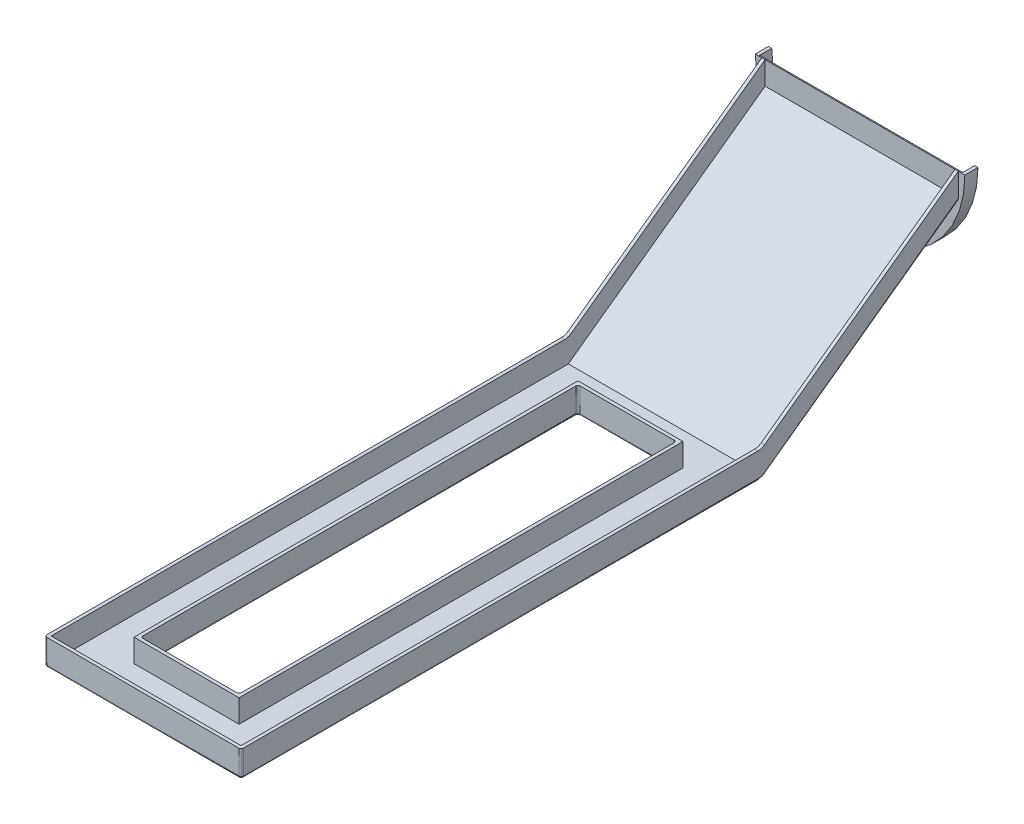
# Autodesk Inventor part: TYLNA SZARA OBUDOWA STOJAKA
Saved by Autodesk Inventor 2017 SP1 (Build 210196100, 196)
## iProperties
Created: 2020-12-26
Part Number: TYLNA SZARA OBUDOWA STOJAKA
Material: Tworzywo sztuczne, nieprzezroczyste czarne
Document SubType Name: Modeling
Designer: Napoleon
Mass: 96.6622 g
Surface Area: 795.491 cm^2
Volume: 101.536 cm^3
Density: 0.952 g/cm^3
Appearance: Teksturowany — drobny — czarny
Author: Napoleon
Autodesk Inventor part; units mm, degrees
ref_plane "YZ Plane" through (0, 0, 0) normal (1, 0, 0) x (0, 1, 0)
sketch "Szkic1" plane through (0, 0, 0) normal (0, 0, 1) x (1, 0, 0)
  line L0 (-44.8776, 28.0247) -> (-44.8776, 13.0664) projected
  arc A0 (-44.8776, 13.0664) -> (-35.2734, -8.1745) centre (0, 20.5664) ccw projected
  arc A1 (-35.2734, -8.1745) -> (-34.8858, -8.3586) centre (-34.8858, -7.8586) ccw projected
  line L1 (-34.8858, -8.3586) -> (-30.8, -8.3586) projected
  arc A2 (-30.3, -8.8586) -> (-30.8, -8.3586) centre (-30.8, -8.8586) ccw projected
  line L2 (-30.3, -8.8586) -> (-30.3, -13.1525) projected
  arc A3 (-30.3, -13.1525) -> (-30.1311, -13.5271) centre (-29.8, -13.1525) ccw projected
  arc A4 (-30.1311, -13.5271) -> (-13.1656, -22.9873) centre (0, 20.5664) ccw projected
  arc A5 (-13.1656, -22.9873) -> (-13.0209, -23.0086) centre (-13.0209, -22.5086) ccw projected
  line L3 (-13.0209, -23.0086) -> (13.0209, -23.0086) projected
  arc A6 (13.0209, -23.0086) -> (13.1656, -22.9873) centre (13.0209, -22.5086) ccw projected
  arc A7 (13.1656, -22.9873) -> (30.1311, -13.5271) centre (0, 20.5664) ccw projected
  arc A8 (30.1311, -13.5271) -> (30.3, -13.1525) centre (29.8, -13.1525) ccw projected
  line L4 (30.3, -13.1525) -> (30.3, -8.8586) projected
  arc A9 (30.8, -8.3586) -> (30.3, -8.8586) centre (30.8, -8.8586) ccw projected
  line L5 (30.8, -8.3586) -> (34.8858, -8.3586) projected
  arc A10 (34.8858, -8.3586) -> (35.2734, -8.1745) centre (34.8858, -7.8586) ccw projected
  arc A11 (35.2734, -8.1745) -> (44.8707, 13.0251) centre (0, 20.5664) ccw projected
  arc A12 (44.8707, 13.0251) -> (44.8776, 13.108) centre (44.3776, 13.108) ccw projected
  line L6 (44.8776, 13.108) -> (44.8776, 28.0247) projected
  arc A13 (44.8776, 28.0247) -> (44.8707, 28.1076) centre (44.3776, 28.0247) ccw projected
  arc A14 (44.8707, 28.1076) -> (35.2734, 49.3072) centre (0, 20.5664) ccw projected
  arc A15 (35.2734, 49.3072) -> (34.8858, 49.4914) centre (34.8858, 48.9914) ccw projected
  line L7 (34.8858, 49.4914) -> (30.8, 49.4914) projected
  arc A16 (30.3, 49.9914) -> (30.8, 49.4914) centre (30.8, 49.9914) ccw projected
  line L8 (30.3, 49.9914) -> (30.3, 54.2852) projected
  arc A17 (30.3, 54.2852) -> (30.1311, 54.6598) centre (29.8, 54.2852) ccw projected
  arc A18 (30.1311, 54.6598) -> (13.1656, 64.12) centre (0, 20.5664) ccw projected
  arc A19 (13.1656, 64.12) -> (13.0209, 64.1414) centre (13.0209, 63.6414) ccw projected
  line L9 (13.0209, 64.1414) -> (-13.0209, 64.1414) projected
  arc A20 (-13.0209, 64.1414) -> (-13.1656, 64.12) centre (-13.0209, 63.6414) ccw projected
  arc A21 (-13.1656, 64.12) -> (-30.1311, 54.6598) centre (0, 20.5664) ccw projected
  arc A22 (-30.1311, 54.6598) -> (-30.3, 54.2852) centre (-29.8, 54.2852) ccw projected
  line L10 (-30.3, 54.2852) -> (-30.3, 49.9914) projected
  arc A23 (-30.8, 49.4914) -> (-30.3, 49.9914) centre (-30.8, 49.9914) ccw projected
  line L11 (-30.8, 49.4914) -> (-34.8858, 49.4914) projected
  arc A24 (-34.8858, 49.4914) -> (-35.2734, 49.3072) centre (-34.8858, 48.9914) ccw projected
  arc A25 (-35.2734, 49.3072) -> (-44.8707, 28.1076) centre (0, 20.5664) ccw projected
  arc A26 (-44.8707, 28.1076) -> (-44.8776, 28.0247) centre (-44.3776, 28.0247) ccw projected
  arc A27 (-47.925, 20.5664) -> (47.925, 20.5664) centre (0, 20.5664) ccw
  line L12 (-47.925, 20.5664) -> (47.925, 20.5664)
  point P0 (0, 0)
  dimension "d0" = 95.85
  constraints: 2 end point, 2 point on circle, 1 centre point, 1 coincident, 1 perpendicular
  measures "d0" diameter of A27
ref_plane "Płaszczyzna konstrukcyjna1" through (-44.8776, -23.0086, -0.5) normal (0, 0, 1) x (1, 0, 0)
extrude "Wyciągnięcie proste1" add sketch "Szkic1" against normal up to surface (0.5 mm away) contours L12 L6 A12 A11 A10 L5 A9 L4 A8 A7 A6 L3 A5 A4 A3 L2 A2 L1 A1 A0 L0 | L0 A0 A1 L1 A2 L2 A3 A4 A5 L3 A6 A7 A8 L4 A9 L5 A10 A11 A12 L6 L12 A27
sketch "Szkic2" plane through (0, 20.5664, -0.5) normal (0, 0, -1) x (-1, 0, 0)
  line L0 (47.925, 0) -> (-47.925, 0) projected
  arc A0 (-47.925, 0) -> (47.925, 0) centre (0, 0) ccw
  arc A1 (-46.425, 0) -> (46.425, 0) centre (0, 0) ccw
  line L1 (47.925, 0) -> (46.425, 0)
  line L2 (-47.925, 0) -> (47.925, 0) projected
  line L3 (-46.425, 0) -> (-47.925, 0)
  point P0 (0, -20.5664)
  dimension "d3" = 92.85
  constraints: 4 end point, 4 point on circle, 2 centre point, 2 collinear, 2 point on line, 1 coincident
  measures "d3" diameter of A1
extrude "Wyciągnięcie proste2" add sketch "Szkic2" along normal blind 5.5 contours A0 L0 A1
sketch "Szkic3" plane through (0, 0, 0) normal (0, 0, 1) x (1, 0, 0)
  arc A0 (-47.925, 20.5664) -> (47.925, 20.5664) centre (0, 20.5664) ccw projected
  line L0 (47.925, 20.5664) -> (-47.925, 20.5664) projected
  line L1 (-46.425, 20.5664) -> (46.425, 20.5664) projected
  line L2 (44.925, 20.5664) -> (44.925, 8.5664)
  line L3 (-44.925, 20.5664) -> (-44.925, 8.5664)
  line L4 (44.925, 8.5664) -> (-44.925, 8.5664)
  line L5 (44.925, 20.5664) -> (43.425, 20.5664)
  line L6 (43.425, 20.5664) -> (43.425, 10.0664)
  line L7 (-44.925, 20.5664) -> (-43.425, 20.5664)
  line L8 (-43.425, 20.5664) -> (-43.425, 10.0664)
  line L9 (43.425, 10.0664) -> (-43.425, 10.0664)
  line L10 (0, 20.5664) -> (0, -44.4336)
  point P0 (0, 0)
  dimension "d8" = 1.5
  dimension "d9" = 10.5
  dimension "d10" = 65
  constraints: 18 end point, 2 horizontal, 2 perpendicular, 2 point on line, 1 vertical
  measures "d8" distance of L2.start L5.end
  measures "d9" distance of L5.end L6.end
  measures "d10" distance of L10.start L10.end
sketch3d "Szkic 3D1"
  line L0 (0, 20.5664, 0) -> (0, -44.4336, 90)
sweep "Przeciągnięcie1" add profiles "Szkic3" path "Szkic 3D1" contours L10 L9 L6 L0 L2 L4 | L4 L3 L0 L8 L9 L10
sketch "Szkic4" plane through (-44.925, -56.4336, 90) normal (0, 0, 1) x (1, 0, 0)
  line L0 (89.85, 12) -> (88.35, 12) projected
  line L1 (88.35, 12) -> (88.35, 1.5) projected
  line L2 (88.35, 1.5) -> (1.5, 1.5) projected
  line L3 (1.5, 1.5) -> (1.5, 12) projected
  line L4 (1.5, 12) -> (0, 12) projected
  line L5 (0, 12) -> (0, 0) projected
  line L6 (0, 0) -> (89.85, 0) projected
  line L7 (89.85, 0) -> (89.85, 12) projected
  point P0 (44.925, 56.4336)
extrude "Wyciągnięcie proste3" add sketch "Szkic4" along normal blind 238
sketch "Szkic5" plane through (-44.925, -56.4336, 90) normal (0, -1, 0) x (1, 0, 0)
  line L0 (88.35, 0) -> (1.5, 0) projected
  line L1 (22.425, 16.5) -> (67.425, 16.5)
  line L2 (67.425, 16.5) -> (67.425, 216.5)
  line L3 (67.425, 216.5) -> (22.425, 216.5)
  line L4 (22.425, 216.5) -> (22.425, 16.5)
  point P0 (44.925, -90)
  dimension "d17" = 45
  dimension "d18" = 200
  constraints: 8 end point, 2 parallel, 1 horizontal, 1 perpendicular
  measures "d17" distance of L3.end L2.end
  measures "d18" distance of L2.end L1.end
extrude "Wyciągnięcie proste4" cut sketch "Szkic5" against normal through all
sketch "Szkic6" plane through (-43.425, -54.9336, 90) normal (0, 1, 0) x (1, 0, 0)
  line L0 (86.85, -238) -> (0, -238) projected
  line L1 (86.85, -238) -> (86.85, -236.5)
  line L2 (86.85, -236.5) -> (0, -236.5)
  line L3 (0, -238) -> (86.85, -238)
  line L4 (0, -238) -> (0, -236.5)
  line L5 (67.425, -218) -> (19.425, -218)
  line L6 (19.425, -218) -> (19.425, -15)
  line L7 (19.425, -15) -> (67.425, -15)
  line L8 (67.425, -15) -> (67.425, -218)
  line L9 (65.925, -16.5) -> (65.925, -216.5)
  line L10 (65.925, -216.5) -> (20.925, -216.5)
  line L11 (20.925, -216.5) -> (20.925, -16.5)
  line L12 (20.925, -16.5) -> (65.925, -16.5)
  point P0 (43.425, 90)
  constraints: 24 end point, 3 equal length, 2 perpendicular, 1 horizontal
extrude "Wyciągnięcie proste5" add sketch "Szkic6" along normal up to surface (10.5 mm away)
fillet "Zaokrąglenie1" radius 1 15 edges at (0, -56.4336, 328) (-44.925, -56.4336, 209) (44.925, -56.4336, 209) (-22.5, -56.4336, 206.5) (22.5, -56.4336, 206.5) (0, -56.4336, 306.5) (0, -56.4336, 106.5) (-22.5, -50.4336, 106.5) (22.5, -50.4336, 106.5) (-22.5, -50.4336, 306.5) (22.5, -50.4336, 306.5) (44.925, -50.4336, 328) (-44.925, -50.4336, 328) (44.925, -23.9336, 45) (-44.925, -23.9336, 45)
fillet "Zaokrąglenie2" radius 5 3 edges at (44.6321, -56.1408, 90.0947) (-44.6321, -56.1408, 90.0947) (0, -56.4336, 90)
sketch "Szkic7" plane through (0, 0, 0) normal (0, 0, 1) x (1, 0, 0)
  arc A0 (-31.75, 8.5664) -> (31.75, 8.5664) centre (0, 9.4024) ccw
  line L0 (-31.75, 8.5664) -> (31.75, 8.5664)
  point P0 (0, 0)
  constraints: 2 end point, 2 point on circle, 1 centre point
sketch3d "Szkic 3D2"
  line L0 (0, -22.3586, 0) -> (0, -45.5337, 74.9078)
sweep "Przeciągnięcie2" add profiles "Szkic7" path "Szkic 3D2"
ref_plane "Płaszczyzna konstrukcyjna2" through (-31.75, 9.7999, 0) normal (-1, 0, 0) x (0, 0, 1)
sketch "Szkic8" plane through (-31.75, 9.7999, 0) normal (-1, 0, 0) x (0, 0, 1)
  line L0 (3.6334, -2.3576) -> (74.9078, -24.4086)
  line L1 (74.9078, -53.8336) -> (74.9078, -24.4086)
  line L2 (3.6334, -2.3576) -> (74.9078, -53.8336)
  point P0 (0, -9.7999)
  constraints: 6 end point
extrude "Wyciągnięcie proste7" cut sketch "Szkic8" against normal blind 63.5
fillet "Zaokrąglenie5" radius 5 2 edges at (44.175, -44.4336, 90) (-44.175, -44.4336, 90)
